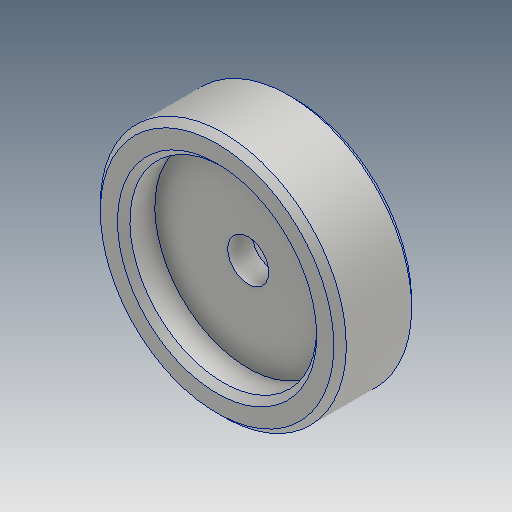
# Autodesk Inventor part: 200-20-ROCKER-CONNECTOR-02
Saved by Autodesk Inventor 2018.2 (Build 222227000, 227)
## iProperties
Manager: feesmrt
Company: FRANC0R
Created: 2017-11-01
Part Number: 200-20-ROCKER-CONNECTOR-02
Material: Aluminium 6061
Document SubType Name: Modeling
Designer: feesmrt
Density: 2.7 g/cm^3
Appearance: Aluminium - flach
Project: Rescue Robot
Cost Center: -
Description: Rocker Profile Connector Fixation
Engineer: feesmrt
Authority: feesmrt
Stock Number: 200-20-ROCKER-CONNECTOR-02
Author: feesmrt
Title: Rocker Profile Connector Fixation
Subject: Rescue Robot
Revision Number: 1
Autodesk Inventor part; units mm, degrees
ref_plane "YZ Plane" through (0, 0, 0) normal (1, 0, 0) x (0, 1, 0)
ref_plane "XZ Plane" through (0, 0, 0) normal (0, 1, 0) x (-1, 0, 0)
ref_plane "XY Plane" through (0, 0, 0) normal (0, 0, 1) x (1, 0, 0)
sketch "Skizze1" plane through (0, 0, 0) normal (1, 0, 0) x (0, 1, 0)
  line L0 (-15, 0) -> (2.5, 0) projected
  line L1 (0, 23.7) -> (0, -3.95) construction
  line L2 (0, 0) -> (0, 19.75)
  line L3 (0, 19.75) -> (-12.5, 19.75)
  line L4 (-12.5, 19.75) -> (-12.5, 15)
  line L5 (-12.5, 15) -> (-7.5, 15)
  line L6 (-7.5, 15) -> (-7.5, 0)
  line L7 (0, 0) -> (-7.5, 0)
  dimension "d0" = 12.5
  dimension "d1" = 39.5
  dimension "d2" = 30
  dimension "d3" = 5
  constraints: 12 end point, 4 perpendicular, 2 point on line, 1 horizontal
  measures "d0" distance of L2.end L3.end
  measures "d1" diameter of L3 L0
  measures "d2" diameter of L5 L0
  measures "d3" distance between parallel lines of L4 L6
revolve "Grundkoerper" add sketch "Skizze1" angle 360 about axis through (0, 0, 0) along (0, 1, 0)
sketch "Skizze2" plane through (0, 0, 0) normal (0, 1, 0) x (1, 0, 0)
  line L0 (0, 27.65) -> (0, -27.65) construction
  line L1 (27.65, 0) -> (-27.65, 0) construction
  point P0 (0, 0)
  point P1 (0, 0)
  constraints: 1 coincident
hole "BOH_M6_ISO10642" at (0, 0, 0) direction (0, -1, 0) diameter 6.6 end through all countersink diameter 13.7 countersink angle 90
chamfer "Fase1" distance 1 angle 45 3 edges at (0, -12.5, -15) (0, -12.5, -19.75) (0, 0, -19.75)
